Autodesk Fusion 360 part; units mm, degrees
(part 4 of 8)
  spline S1001 degree 3 poles (12.7984, -90.8958) (12.7866, -90.9224) (12.7444, -90.9476) (12.7042, -90.9476) knots 0 0 0 0 1 1 1 1
  spline S1002 degree 3 poles (12.7042, -90.9476) (12.6392, -90.9505) (12.642, -90.9527) (12.7088, -90.9646) knots 0 0 0 0 1 1 1 1
  spline S1003 degree 3 poles (14.8306, -88.329) (14.8946, -88.3388) (14.9475, -88.3398) (14.9491, -88.3321) knots 0 0 0 0 1 1 1 1
  spline S1004 degree 3 poles (14.9491, -88.3321) (14.9427, -88.3002) (14.7543, -88.2605) (14.7348, -88.2855) knots 0 0 0 0 1 1 1 1
  spline S1005 degree 3 poles (14.7348, -88.2855) (14.7218, -88.3022) (14.7666, -88.3193) (14.8306, -88.329) knots 0 0 0 0 1 1 1 1
  spline S1006 degree 3 poles (4.5302, -101.5016) (4.5488, -101.4892) (4.5748, -101.4559) (4.5845, -101.4321) knots 0 0 0 0 1 1 1 1
  spline S1007 degree 3 poles (4.5845, -101.4321) (4.5892, -101.4089) (4.5727, -101.4184) (4.5423, -101.4573) knots 0 0 0 0 1 1 1 1
  spline S1008 degree 3 poles (4.5423, -101.4573) (4.5119, -101.4963) (4.5066, -101.5145) (4.5302, -101.5016) knots 0 0 0 0 1 1 1 1
  spline S1009 degree 3 poles (11.2167, -93.0176) (11.2886, -92.9887) (11.3694, -92.931) (11.3998, -92.8921) knots 0 0 0 0 1 1 1 1
  spline S1010 degree 3 poles (11.3998, -92.8921) (11.4346, -92.8476) (11.3962, -92.8624) (11.2819, -92.9343) knots 0 0 0 0 1 1 1 1
  spline S1011 degree 3 poles (11.2819, -92.9343) (11.0653, -93.0739) (11.0544, -93.0878) (11.2167, -93.0176) knots 0 0 0 0 1 1 1 1
  spline S1012 degree 3 poles (12.0049, -91.9859) (11.9836, -92.0991) (12.0323, -92.1686) (12.1069, -92.1418) knots 0 0 0 0 1 1 1 1
  spline S1013 degree 3 poles (12.1069, -92.1418) (12.1333, -92.131) (12.1265, -92.1168) (12.0817, -92.0997) knots 0 0 0 0 1 1 1 1
  spline S1014 degree 3 poles (12.0817, -92.0997) (12.0291, -92.081) (12.0199, -92.0469) (12.038, -91.9492) knots 0 0 0 0 1 1 1 1
  spline S1015 degree 3 poles (12.038, -91.9492) (12.0549, -91.8818) (12.0566, -91.8338) (12.0435, -91.8505) knots 0 0 0 0 1 1 1 1
  spline S1016 degree 3 poles (12.0435, -91.8505) (12.0327, -91.8644) (12.0152, -91.9269) (12.0049, -91.9859) knots 0 0 0 0 1 1 1 1
  spline S1017 degree 3 poles (14.5723, -88.7227) (14.5927, -88.7252) (14.6175, -88.7221) (14.624, -88.7138) knots 0 0 0 0 1 1 1 1
  spline S1018 degree 3 poles (14.624, -88.7138) (14.6284, -88.7082) (14.6188, -88.6918) (14.6049, -88.681) knots 0 0 0 0 1 1 1 1
  spline S1019 degree 3 poles (14.6049, -88.681) (14.5882, -88.6679) (14.5662, -88.6731) (14.5532, -88.6898) knots 0 0 0 0 1 1 1 1
  spline S1020 degree 3 poles (14.5532, -88.6898) (14.5424, -88.7037) (14.5491, -88.718) (14.5723, -88.7227) knots 0 0 0 0 1 1 1 1
  spline S1021 degree 3 poles (4.281, -101.9695) (4.306, -101.989) (4.5908, -102.0772) (4.9108, -102.1661) knots 0 0 0 0 1 1 1 1
  spline S1022 degree 3 poles (4.9108, -102.1661) (5.4408, -102.3071) (5.533, -102.3209) (5.9897, -102.3151) knots 0 0 0 0 1 1 1 1
  line L78 (5.9897, -102.3151) -> (6.486, -102.3044)
  line L79 (6.486, -102.3044) -> (6.739, -102.502)
  line L80 (6.739, -102.502) -> (6.9892, -102.6975)
  line L81 (6.9892, -102.6975) -> (6.99, -105.5902)
  spline S1023 degree 3 poles (6.99, -105.5902) (6.9896, -107.1836) (6.9897, -108.5759) (6.9888, -108.6917) knots 0 0 0 0 1 1 1 1
  spline S1024 degree 3 poles (6.9888, -108.6917) (6.9873, -108.8024) (6.9877, -109.5011) (6.9879, -110.2399) knots 0 0 0 0 1 1 1 1
  spline S1025 degree 3 poles (6.9879, -110.2399) (6.9881, -110.9788) (6.991, -112.0868) (6.9887, -112.7028) knots 0 0 0 0 1 1 1 1
  spline S1026 degree 3 poles (6.9887, -112.7028) (6.9874, -115.455) (6.9879, -117.179) (6.9875, -118.3427) knots 0 0 0 0 1 1 1 1
  spline S1027 degree 3 poles (6.9875, -118.3427) (6.9869, -119.7703) (6.9887, -121.7907) (6.9896, -123.7836) knots 0 0 0 0 1 1 1 1
  spline S1028 degree 3 poles (6.9896, -123.7836) (6.9889, -124.5352) (6.9928, -125.1605) (7.0002, -125.1797) knots 0 0 0 0 1 1 1 1
  spline S1029 degree 3 poles (7.0002, -125.1797) (7.0128, -125.2209) (8.7969, -126.467) (8.9109, -126.5159) knots 0 0 0 0 1 1 1 1
  spline S1030 degree 3 poles (8.9109, -126.5159) (9.0544, -126.5787) (9.3568, -126.3807) (9.4107, -126.1856) knots 0 0 0 0 1 1 1 1
  spline S1031 degree 3 poles (9.4107, -126.1856) (9.4357, -126.1021) (9.4813, -126.0437) (9.6313, -125.9147) knots 0 0 0 0 1 1 1 1
  spline S1032 degree 3 poles (9.6313, -125.9147) (9.7355, -125.8215) (9.9286, -125.6545) (10.0551, -125.5385) knots 0 0 0 0 1 1 1 1
  spline S1033 degree 3 poles (10.0551, -125.5385) (10.2253, -125.3894) (10.2996, -125.3401) (10.3188, -125.3729) knots 0 0 0 0 1 1 1 1
  spline S1034 degree 3 poles (10.3188, -125.3729) (10.3502, -125.4243) (10.3645, -125.4175) (10.761, -125.0648) knots 0 0 0 0 1 1 1 1
  spline S1035 degree 3 poles (10.761, -125.0648) (11.0756, -124.7823) (11.1153, -124.7373) (11.2557, -124.4888) knots 0 0 0 0 1 1 1 1
  spline S1036 degree 3 poles (11.2557, -124.4888) (11.3514, -124.3263) (11.4189, -124.1596) (11.4315, -124.0576) knots 0 0 0 0 1 1 1 1
  spline S1037 degree 3 poles (11.4315, -124.0576) (11.4484, -123.9499) (11.5203, -123.7777) (11.6461, -123.5537) knots 0 0 0 0 1 1 1 1
  spline S1038 degree 3 poles (11.6461, -123.5537) (11.8113, -123.262) (11.8911, -123.1542) (12.2332, -122.7678) knots 0 0 0 0 1 1 1 1
  spline S1039 degree 3 poles (12.2332, -122.7678) (12.651, -122.3019) (12.7087, -122.1993) (12.6499, -122.0683) knots 0 0 0 0 1 1 1 1
  spline S1040 degree 3 poles (12.6499, -122.0683) (12.6364, -122.0398) (12.4699, -121.7485) (12.2816, -121.4223) knots 0 0 0 0 1 1 1 1
  spline S1041 degree 3 poles (12.2816, -121.4223) (12.0933, -121.0961) (11.9333, -120.7966) (11.9306, -120.7542) knots 0 0 0 0 1 1 1 1
  spline S1042 degree 3 poles (11.9306, -120.7542) (11.9279, -120.7118) (11.9034, -120.6344) (11.8763, -120.5774) knots 0 0 0 0 1 1 1 1
  spline S1043 degree 3 poles (11.8763, -120.5774) (11.8073, -120.425) (11.7691, -119.9296) (11.8234, -119.8601) knots 0 0 0 0 1 1 1 1
  spline S1044 degree 3 poles (11.8234, -119.8601) (11.8473, -119.8295) (12.0503, -119.6613) (12.2682, -119.4913) knots 0 0 0 0 1 1 1 1
  spline S1045 degree 3 poles (12.2682, -119.4913) (12.4861, -119.3213) (12.6847, -119.1587) (12.7086, -119.1281) knots 0 0 0 0 1 1 1 1
  spline S1046 degree 3 poles (12.7086, -119.1281) (12.7499, -119.0753) (12.7349, -118.871) (12.6848, -118.8319) knots 0 0 0 0 1 1 1 1
  spline S1047 degree 3 poles (12.6848, -118.8319) (12.6292, -118.7885) (12.0506, -117.8216) (12.0208, -117.7222) knots 0 0 0 0 1 1 1 1
  spline S1048 degree 3 poles (12.0208, -117.7222) (11.9944, -117.6299) (12.0202, -117.574) (12.3693, -116.9782) knots 0 0 0 0 1 1 1 1
  spline S1049 degree 3 poles (12.3693, -116.9782) (12.5773, -116.6259) (12.7532, -116.2977) (12.7604, -116.2541) knots 0 0 0 0 1 1 1 1
  spline S1050 degree 3 poles (12.7604, -116.2541) (12.7698, -116.2077) (12.7483, -116.1148) (12.7138, -116.0387) knots 0 0 0 0 1 1 1 1
  spline S1051 degree 3 poles (12.7138, -116.0387) (12.6217, -115.8414) (11.9083, -114.5542) (11.8777, -114.5303) knots 0 0 0 0 1 1 1 1
  spline S1052 degree 3 poles (11.8777, -114.5303) (11.8332, -114.4956) (11.8403, -114.3489) (11.8999, -113.9747) knots 0 0 0 0 1 1 1 1
  spline S1053 degree 3 poles (11.8999, -113.9747) (11.936, -113.7566) (11.9912, -113.5714) (12.0303, -113.5214) knots 0 0 0 0 1 1 1 1
  spline S1054 degree 3 poles (12.0303, -113.5214) (12.0672, -113.4741) (12.3083, -113.3088) (12.5611, -113.1571) knots 0 0 0 0 1 1 1 1
  spline S1055 degree 3 poles (12.5611, -113.1571) (12.8161, -113.0027) (13.0419, -112.8568) (13.0637, -112.829) knots 0 0 0 0 1 1 1 1
  spline S1056 degree 3 poles (13.0637, -112.829) (13.1223, -112.754) (13.1248, -112.5903) (13.0742, -112.1165) knots 0 0 0 0 1 1 1 1
  line L82 (13.0742, -112.1165) -> (13.0312, -111.6844)
  line L83 (13.0312, -111.6844) -> (12.759, -111.2077)
  spline S1057 degree 3 poles (12.759, -111.2077) (12.4924, -110.7352) (12.489, -110.7281) (12.4214, -110.2589) knots 0 0 0 0 1 1 1 1
  spline S1058 degree 3 poles (12.4214, -110.2589) (12.3842, -109.9971) (12.3686, -109.7477) (12.3885, -109.705) knots 0 0 0 0 1 1 1 1
  spline S1059 degree 3 poles (12.3885, -109.705) (12.41, -109.6546) (12.5476, -109.5472) (12.7505, -109.4193) knots 0 0 0 0 1 1 1 1
  spline S1060 degree 3 poles (12.7505, -109.4193) (13.1329, -109.1763) (13.1565, -109.1231) (13.0008, -108.8985) knots 0 0 0 0 1 1 1 1
  spline S1061 degree 3 poles (13.0008, -108.8985) (12.9486, -108.8219) (12.7984, -108.6016) (12.6667, -108.4092) knots 0 0 0 0 1 1 1 1
  spline S1062 degree 3 poles (12.6667, -108.4092) (12.5329, -108.2195) (12.4166, -108.0302) (12.4068, -107.9912) knots 0 0 0 0 1 1 1 1
  spline S1063 degree 3 poles (12.4068, -107.9912) (12.3832, -107.9011) (12.3853, -106.6493) (12.4092, -106.6187) knots 0 0 0 0 1 1 1 1
  spline S1064 degree 3 poles (12.4092, -106.6187) (12.4179, -106.6076) (12.442, -106.5996) (12.4603, -106.6049) knots 0 0 0 0 1 1 1 1
  spline S1065 degree 3 poles (12.4603, -106.6049) (12.5206, -106.6251) (13.1255, -106.6187) (13.1428, -106.5965) knots 0 0 0 0 1 1 1 1
  spline S1066 degree 3 poles (13.1428, -106.5965) (13.1581, -106.577) (13.1685, -105.4749) (13.1578, -104.4458) knots 0 0 0 0 1 1 1 1
  spline S1067 degree 3 poles (13.1578, -104.4458) (13.159, -104.1692) (13.1651, -103.9322) (13.1781, -103.9155) knots 0 0 0 0 1 1 1 1
  spline S1068 degree 3 poles (13.1781, -103.9155) (13.1911, -103.8989) (13.2019, -103.6387) (13.2023, -103.3345) knots 0 0 0 0 1 1 1 1
  spline S1069 degree 3 poles (13.2023, -103.3345) (13.1977, -103.031) (13.2023, -102.7615) (13.1992, -102.7367) knots 0 0 0 0 1 1 1 1
  spline S1070 degree 3 poles (13.1992, -102.7367) (13.2015, -102.6937) (13.5834, -102.3654) (13.6673, -102.3324) knots 0 0 0 0 1 1 1 1
  spline S1071 degree 3 poles (13.6673, -102.3324) (13.6915, -102.3245) (13.9245, -102.3185) (14.1862, -102.3215) knots 0 0 0 0 1 1 1 1
  spline S1072 degree 3 poles (14.1862, -102.3215) (14.6067, -102.3277) (14.7228, -102.3109) (15.2748, -102.1602) knots 0 0 0 0 1 1 1 1
  spline S1073 degree 3 poles (15.2748, -102.1602) (15.6125, -102.066) (15.9073, -101.9694) (15.9241, -101.9423) knots 0 0 0 0 1 1 1 1
  spline S1074 degree 3 poles (15.9241, -101.9423) (15.9545, -101.9033) (15.9489, -101.899) (15.9117, -101.9237) knots 0 0 0 0 1 1 1 1
  spline S1075 degree 3 poles (15.9117, -101.9237) (15.8832, -101.9372) (15.6092, -102.0186) (15.2956, -102.1049) knots 0 0 0 0 1 1 1 1
  spline S1076 degree 3 poles (15.2956, -102.1049) (14.804, -102.2356) (14.6632, -102.2554) (14.2136, -102.2578) knots 0 0 0 0 1 1 1 1
  spline S1077 degree 3 poles (14.2136, -102.2578) (13.7436, -102.2577) (13.5797, -102.2326) (13.7682, -102.1919) knots 0 0 0 0 1 1 1 1
  spline S1078 degree 3 poles (13.7682, -102.1919) (13.8391, -102.1756) (13.8363, -102.1735) (13.7546, -102.1634) knots 0 0 0 0 1 1 1 1
  spline S1079 degree 3 poles (13.7546, -102.1634) (13.6863, -102.1592) (13.6649, -102.1694) (13.6654, -102.2146) knots 0 0 0 0 1 1 1 1
  spline S1080 degree 3 poles (13.6654, -102.2146) (13.6668, -102.2873) (13.2945, -102.5918) (13.1769, -102.6163) knots 0 0 0 0 1 1 1 1
  spline S1081 degree 3 poles (13.1769, -102.6163) (13.1104, -102.627) (13.1001, -102.6459) (13.107, -102.7632) knots 0 0 0 0 1 1 1 1
  spline S1082 degree 3 poles (13.107, -102.7632) (13.1289, -103.0847) (13.111, -103.8811) (13.0881, -103.8989) knots 0 0 0 0 1 1 1 1
  spline S1083 degree 3 poles (13.0881, -103.8989) (13.0695, -103.9113) (13.0342, -103.9106) (13.0055, -103.9016) knots 0 0 0 0 1 1 1 1
  spline S1084 degree 3 poles (13.0055, -103.9016) (12.9634, -103.8866) (12.9699, -103.8783) (13.0408, -103.862) knots 0 0 0 0 1 1 1 1
  spline S1085 degree 3 poles (13.0408, -103.862) (13.1188, -103.8424) (13.1188, -103.8424) (13.0461, -103.8438) knots 0 0 0 0 1 1 1 1
  spline S1086 degree 3 poles (13.0461, -103.8438) (13.0031, -103.8415) (12.9675, -103.8585) (12.9622, -103.8767) knots 0 0 0 0 1 1 1 1
  spline S1087 degree 3 poles (12.9622, -103.8767) (12.9619, -103.8943) (12.5995, -103.9112) (12.1592, -103.9074) knots 0 0 0 0 1 1 1 1
  spline S1088 degree 3 poles (12.1592, -103.9074) (11.7168, -103.9065) (11.3566, -103.9205) (11.3569, -103.9431) knots 0 0 0 0 1 1 1 1
  spline S1089 degree 3 poles (11.3569, -103.9431) (11.3593, -103.9629) (11.351, -103.9564) (11.3402, -103.9301) knots 0 0 0 0 1 1 1 1
  spline S1090 degree 3 poles (11.3402, -103.9301) (11.3226, -103.8895) (11.3384, -103.875) (11.4149, -103.8631) knots 0 0 0 0 1 1 1 1
  spline S1091 degree 3 poles (11.4149, -103.8631) (11.5084, -103.8466) (11.5078, -103.8417) (11.4311, -103.831) knots 0 0 0 0 1 1 1 1
  spline S1092 degree 3 poles (11.4311, -103.831) (11.3896, -103.821) (11.3048, -103.8264) (11.2482, -103.8358) knots 0 0 0 0 1 1 1 1
  spline S1093 degree 3 poles (11.2482, -103.8358) (11.1575, -103.8545) (11.1553, -103.8573) (11.2231, -103.8565) knots 0 0 0 0 1 1 1 1
  spline S1094 degree 3 poles (11.2231, -103.8565) (11.2936, -103.8579) (11.3047, -103.8666) (11.2981, -103.9152) knots 0 0 0 0 1 1 1 1
  spline S1095 degree 3 poles (11.2981, -103.9152) (11.2947, -103.9483) (11.2807, -103.9776) (11.2686, -103.9816) knots 0 0 0 0 1 1 1 1
  spline S1096 degree 3 poles (11.2686, -103.9816) (11.2543, -103.9884) (11.259, -104.0054) (11.2812, -104.0228) knots 0 0 0 0 1 1 1 1
  spline S1097 degree 3 poles (11.2812, -104.0228) (11.3034, -104.0402) (11.3232, -104.0377) (11.3258, -104.0173) knots 0 0 0 0 1 1 1 1
  spline S1098 degree 3 poles (11.3258, -104.0173) (11.3261, -103.9997) (11.3404, -103.9929) (11.3543, -104.0038) knots 0 0 0 0 1 1 1 1
  spline S1099 degree 3 poles (11.3543, -104.0038) (11.3682, -104.0146) (11.3806, -104.1363) (11.3794, -104.2696) knots 0 0 0 0 1 1 1 1
  spline S1100 degree 3 poles (11.3794, -104.2696) (11.3767, -104.4735) (11.3646, -104.5177) (11.3107, -104.5294) knots 0 0 0 0 1 1 1 1
  spline S1101 degree 3 poles (11.3107, -104.5294) (11.264, -104.5376) (11.2531, -104.5515) (11.2754, -104.5689) knots 0 0 0 0 1 1 1 1
  spline S1102 degree 3 poles (11.2754, -104.5689) (11.292, -104.5819) (11.3168, -104.5789) (11.3298, -104.5622) knots 0 0 0 0 1 1 1 1
  spline S1103 degree 3 poles (11.3298, -104.5622) (11.3841, -104.4927) (11.3825, -104.2541) (11.3803, -109.6604) knots 0 0 0 0 1 1 1 1
  spline S1104 degree 3 poles (11.3803, -109.6604) (11.378, -111.136) (11.3595, -112.1109) (11.3328, -112.1393) knots 0 0 0 0 1 1 1 1
  spline S1105 degree 3 poles (11.3328, -112.1393) (11.3033, -112.1655) (11.3036, -112.1881) (11.3324, -112.1971) knots 0 0 0 0 1 1 1 1
  spline S1106 degree 3 poles (11.3324, -112.1971) (11.3611, -112.2062) (11.3792, -112.7217) (11.3792, -113.541) knots 0 0 0 0 1 1 1 1
  line L84 (11.3792, -113.541) -> (11.3813, -114.8677)
  line L85 (11.3813, -114.8677) -> (11.2739, -114.8734)
  line L86 (11.2739, -114.8734) -> (11.1715, -114.8784)
  line L87 (11.1715, -114.8784) -> (11.2736, -114.891)
  spline S1107 degree 3 poles (11.2736, -114.891) (11.3729, -114.9014) (11.379, -114.9107) (11.3784, -115.049) knots 0 0 0 0 1 1 1 1
  spline S1108 degree 3 poles (11.3784, -115.049) (11.3782, -115.1295) (11.3789, -115.6672) (11.3795, -116.2452) knots 0 0 0 0 1 1 1 1
  spline S1109 degree 3 poles (11.3795, -116.2452) (11.3773, -116.821) (11.3759, -117.3213) (11.3796, -117.351) knots 0 0 0 0 1 1 1 1
  spline S1110 degree 3 poles (11.3796, -117.351) (11.3767, -117.3891) (11.3522, -117.4147) (11.3033, -117.4257) knots 0 0 0 0 1 1 1 1
  spline S1111 degree 3 poles (11.3033, -117.4257) (11.2324, -117.442) (11.233, -117.4469) (11.3008, -117.4462) knots 0 0 0 0 1 1 1 1
  spline S1112 degree 3 poles (11.3008, -117.4462) (11.3834, -117.4436) (11.3849, -117.4761) (11.3791, -118.9847) knots 0 0 0 0 1 1 1 1
  spline S1113 degree 3 poles (11.3791, -118.9847) (11.377, -119.6635) (11.3693, -119.8052) (11.33, -119.6492) knots 0 0 0 0 1 1 1 1
  spline S1114 degree 3 poles (11.33, -119.6492) (11.3184, -119.5953) (11.3122, -119.5861) (11.3072, -119.6269) knots 0 0 0 0 1 1 1 1
  spline S1115 degree 3 poles (11.3072, -119.6269) (11.3031, -119.655) (11.2693, -119.6868) (11.2275, -119.6945) knots 0 0 0 0 1 1 1 1
  spline S1116 degree 3 poles (11.2275, -119.6945) (11.1665, -119.7095) (11.1693, -119.7117) (11.2658, -119.7199) knots 0 0 0 0 1 1 1 1
  spline S1117 degree 3 poles (11.2658, -119.7199) (11.3982, -119.7338) (11.3837, -119.5748) (11.3812, -121.171) knots 0 0 0 0 1 1 1 1
  spline S1118 degree 3 poles (11.3812, -121.171) (11.379, -121.7468) (11.3803, -122.2493) (11.3796, -122.2845) knots 0 0 0 0 1 1 1 1
  spline S1119 degree 3 poles (11.3796, -122.2845) (11.3786, -122.3374) (11.3737, -122.3381) (11.3456, -122.2937) knots 0 0 0 0 1 1 1 1
  spline S1120 degree 3 poles (11.3456, -122.2937) (11.3209, -122.2566) (11.3082, -122.2556) (11.2955, -122.2949) knots 0 0 0 0 1 1 1 1
  spline S1121 degree 3 poles (11.2955, -122.2949) (11.2864, -122.3236) (11.3006, -122.3571) (11.3278, -122.3738) knots 0 0 0 0 1 1 1 1
  spline S1122 degree 3 poles (11.3278, -122.3738) (11.376, -122.3981) (11.3855, -122.701) (11.3735, -123.7078) knots 0 0 0 0 1 1 1 1
  spline S1123 degree 3 poles (11.3735, -123.7078) (11.3706, -124.0324) (11.3542, -124.145) (11.2887, -124.246) knots 0 0 0 0 1 1 1 1
  spline S1124 degree 3 poles (11.2887, -124.246) (11.2471, -124.3164) (11.172, -124.4413) (11.1223, -124.5278) knots 0 0 0 0 1 1 1 1
  spline S1125 degree 3 poles (11.1223, -124.5278) (11.0338, -124.687) (10.5314, -125.1809) (10.4119, -125.2308) knots 0 0 0 0 1 1 1 1
  spline S1126 degree 3 poles (10.4119, -125.2308) (10.3664, -125.2489) (10.3553, -125.0568) (10.359, -124.3702) knots 0 0 0 0 1 1 1 1
  spline S1127 degree 3 poles (10.359, -124.3702) (10.3595, -123.8826) (10.3618, -123.2263) (10.3609, -122.9123) knots 0 0 0 0 1 1 1 1
  spline S1128 degree 3 poles (10.3609, -122.9123) (10.3629, -122.4571) (10.3786, -122.3396) (10.4244, -122.344) knots 0 0 0 0 1 1 1 1
  spline S1129 degree 3 poles (10.4244, -122.344) (10.4723, -122.3457) (10.4717, -122.3407) (10.4257, -122.3137) knots 0 0 0 0 1 1 1 1
  spline S1130 degree 3 poles (10.4257, -122.3137) (10.3796, -122.2867) (10.3639, -121.688) (10.364, -119.6824) knots 0 0 0 0 1 1 1 1
  spline S1131 degree 3 poles (10.364, -119.6824) (10.3625, -115.1059) (10.3617, -114.8949) (10.4038, -114.9099) knots 0 0 0 0 1 1 1 1
  spline S1132 degree 3 poles (10.4038, -114.9099) (10.4591, -114.9307) (10.484, -114.8874) (10.4497, -114.8338) knots 0 0 0 0 1 1 1 1
  spline S1133 degree 3 poles (10.4497, -114.8338) (10.4278, -114.7988) (10.4158, -114.8028) (10.4008, -114.8449) knots 0 0 0 0 1 1 1 1
  spline S1134 degree 3 poles (10.4008, -114.8449) (10.3821, -114.8974) (10.3794, -114.8953) (10.3715, -114.8309) knots 0 0 0 0 1 1 1 1
  spline S1135 degree 3 poles (10.3715, -114.8309) (10.3401, -114.596) (10.3688, -112.2099) (10.4017, -112.1908) knots 0 0 0 0 1 1 1 1
  spline S1136 degree 3 poles (10.4017, -112.1908) (10.4224, -112.1757) (10.425, -112.1552) (10.4033, -112.1428) knots 0 0 0 0 1 1 1 1
  spline S1137 degree 3 poles (10.4033, -112.1428) (10.3811, -112.1254) (10.364, -111.454) (10.363, -110.6474) knots 0 0 0 0 1 1 1 1
  line L88 (10.363, -110.6474) -> (10.3609, -109.1774)
  line L89 (10.3609, -109.1774) -> (10.4683, -109.1717)
  line L90 (10.4683, -109.1717) -> (10.5757, -109.1661)
  line L91 (10.5757, -109.1661) -> (10.4686, -109.1541)
  line L92 (10.4686, -109.1541) -> (10.3638, -109.1393)
  line L93 (10.3638, -109.1393) -> (10.3631, -107.8853)
  spline S1138 degree 3 poles (10.3631, -107.8853) (10.3634, -107.1916) (10.3826, -106.6112) (10.3978, -106.5917) knots 0 0 0 0 1 1 1 1
  spline S1139 degree 3 poles (10.3978, -106.5917) (10.418, -106.5717) (10.4177, -106.5491) (10.3988, -106.5388) knots 0 0 0 0 1 1 1 1
  spline S1140 degree 3 poles (10.3988, -106.5388) (10.3828, -106.5307) (10.3661, -106.0879) (10.3639, -105.5579) knots 0 0 0 0 1 1 1 1
  spline S1141 degree 3 poles (10.3639, -105.5579) (10.3642, -104.9673) (10.3449, -104.5851) (10.3156, -104.5711) knots 0 0 0 0 1 1 1 1
  spline S1142 degree 3 poles (10.3156, -104.5711) (10.289, -104.5593) (10.2782, -104.533) (10.2912, -104.5163) knots 0 0 0 0 1 1 1 1
  spline S1143 degree 3 poles (10.2912, -104.5163) (10.3043, -104.4996) (10.3197, -104.5028) (10.3299, -104.5241) knots 0 0 0 0 1 1 1 1
  spline S1144 degree 3 poles (10.3299, -104.5241) (10.3373, -104.5433) (10.3555, -104.5486) (10.3664, -104.5347) knots 0 0 0 0 1 1 1 1
  spline S1145 degree 3 poles (10.3664, -104.5347) (10.3794, -104.518) (10.4042, -104.515) (10.4209, -104.528) knots 0 0 0 0 1 1 1 1
  spline S1146 degree 3 poles (10.4209, -104.528) (10.4348, -104.5389) (10.4344, -104.5565) (10.4152, -104.5639) knots 0 0 0 0 1 1 1 1
  spline S1147 degree 3 poles (10.4152, -104.5639) (10.3356, -104.5913) (10.4401, -104.6639) (10.5335, -104.6474) knots 0 0 0 0 1 1 1 1
  spline S1148 degree 3 poles (10.5335, -104.6474) (10.6314, -104.6253) (10.6314, -104.6253) (10.5339, -104.6298) knots 0 0 0 0 1 1 1 1
  spline S1149 degree 3 poles (10.5339, -104.6298) (10.4463, -104.633) (10.438, -104.6265) (10.4545, -104.5767) knots 0 0 0 0 1 1 1 1
  spline S1150 degree 3 poles (10.4545, -104.5767) (10.4794, -104.4932) (10.4269, -104.4745) (10.226, -104.4967) knots 0 0 0 0 1 1 1 1
  spline S1151 degree 3 poles (10.226, -104.4967) (10.127, -104.5088) (10.0901, -104.5159) (10.148, -104.5163) knots 0 0 0 0 1 1 1 1
  spline S1152 degree 3 poles (10.148, -104.5163) (10.2031, -104.5146) (10.2522, -104.5261) (10.2541, -104.541) knots 0 0 0 0 1 1 1 1
  spline S1153 degree 3 poles (10.2541, -104.541) (10.2559, -104.5558) (10.0841, -104.5694) (9.8753, -104.5674) knots 0 0 0 0 1 1 1 1
  spline S1154 degree 3 poles (9.8753, -104.5674) (9.5965, -104.5689) (9.4876, -104.5823) (9.4705, -104.6271) knots 0 0 0 0 1 1 1 1
  spline S1155 degree 3 poles (9.4705, -104.6271) (9.454, -104.6769) (9.449, -104.6775) (9.4522, -104.6218) knots 0 0 0 0 1 1 1 1
  spline S1156 degree 3 poles (9.4522, -104.6218) (9.456, -104.5711) (9.4421, -104.5602) (9.3926, -104.5663) knots 0 0 0 0 1 1 1 1
  spline S1157 degree 3 poles (9.3926, -104.5663) (9.3629, -104.57) (9.3221, -104.5649) (9.3082, -104.5541) knots 0 0 0 0 1 1 1 1
  spline S1158 degree 3 poles (9.3082, -104.5541) (9.2943, -104.5432) (9.3652, -104.527) (9.467, -104.517) knots 0 0 0 0 1 1 1 1
  spline S1159 degree 3 poles (9.467, -104.517) (9.5716, -104.5092) (9.6029, -104.4978) (9.5422, -104.4952) knots 0 0 0 0 1 1 1 1
  spline S1160 degree 3 poles (9.5422, -104.4952) (9.4766, -104.4932) (9.3878, -104.4865) (9.3399, -104.4848) knots 0 0 0 0 1 1 1 1
  spline S1161 degree 3 poles (9.3399, -104.4848) (9.2638, -104.4791) (9.2551, -104.4902) (9.2602, -104.5524) knots 0 0 0 0 1 1 1 1
  spline S1162 degree 3 poles (9.2602, -104.5524) (9.2675, -104.6118) (9.2567, -104.6257) (9.2006, -104.6402) knots 0 0 0 0 1 1 1 1
  spline S1163 degree 3 poles (9.2006, -104.6402) (9.1369, -104.653) (9.1396, -104.6552) (9.2235, -104.6625) knots 0 0 0 0 1 1 1 1
  spline S1164 degree 3 poles (9.2235, -104.6625) (9.2875, -104.6722) (9.311, -104.6593) (9.2969, -104.6258) knots 0 0 0 0 1 1 1 1
  spline S1165 degree 3 poles (9.2969, -104.6258) (9.2849, -104.5896) (9.2892, -104.584) (9.3143, -104.6036) knots 0 0 0 0 1 1 1 1
  spline S1166 degree 3 poles (9.3143, -104.6036) (9.3337, -104.6188) (9.3498, -105.0566) (9.3486, -105.5795) knots 0 0 0 0 1 1 1 1
  line L94 (9.3486, -105.5795) -> (9.3518, -106.5266)
  line L95 (9.3518, -106.5266) -> (9.2088, -106.5492)
  line L96 (9.2088, -106.5492) -> (9.0658, -106.5718)
  line L97 (9.0658, -106.5718) -> (9.2075, -106.5795)
  spline S1167 degree 3 poles (9.2075, -106.5795) (9.2929, -106.5791) (9.3483, -106.6) (9.3519, -106.6297) knots 0 0 0 0 1 1 1 1
  spline S1168 degree 3 poles (9.3519, -106.6297) (9.3522, -106.6523) (9.3516, -107.2203) (9.3532, -107.8887) knots 0 0 0 0 1 1 1 1
  spline S1169 degree 3 poles (9.3532, -107.8887) (9.35, -108.9069) (9.3375, -109.112) (9.2827, -109.1363) knots 0 0 0 0 1 1 1 1
  spline S1170 degree 3 poles (9.2827, -109.1363) (9.2328, -109.1601) (9.2248, -109.1761) (9.2526, -109.1978) knots 0 0 0 0 1 1 1 1
  spline S1171 degree 3 poles (9.2526, -109.1978) (9.2748, -109.2152) (9.2946, -109.2128) (9.2971, -109.1924) knots 0 0 0 0 1 1 1 1
  spline S1172 degree 3 poles (9.2971, -109.1924) (9.2975, -109.1747) (9.3117, -109.168) (9.3256, -109.1788) knots 0 0 0 0 1 1 1 1
  spline S1173 degree 3 poles (9.3256, -109.1788) (9.3451, -109.194) (9.3588, -110.8611) (9.3473, -111.8729) knots 0 0 0 0 1 1 1 1
  spline S1174 degree 3 poles (9.3473, -111.8729) (9.3448, -112.1396) (9.3417, -112.155) (9.2613, -112.1549) knots 0 0 0 0 1 1 1 1
  spline S1175 degree 3 poles (9.2613, -112.1549) (9.1836, -112.1569) (9.1836, -112.1569) (9.2637, -112.1747) knots 0 0 0 0 1 1 1 1
  spline S1176 degree 3 poles (9.2637, -112.1747) (9.3438, -112.1925) (9.3487, -112.2321) (9.3495, -112.6894) knots 0 0 0 0 1 1 1 1
  spline S1177 degree 3 poles (9.3495, -112.6894) (9.3526, -112.9605) (9.3701, -113.1845) (9.3955, -113.1864) knots 0 0 0 0 1 1 1 1
  spline S1178 degree 3 poles (9.3955, -113.1864) (9.4187, -113.1911) (9.4171, -113.1988) (9.3929, -113.2068) knots 0 0 0 0 1 1 1 1
  spline S1179 degree 3 poles (9.3929, -113.2068) (9.3688, -113.2148) (9.3504, -113.5765) (9.3506, -114.0288) knots 0 0 0 0 1 1 1 1
  spline S1180 degree 3 poles (9.3506, -114.0288) (9.3496, -114.798) (9.3393, -114.9601) (9.3016, -114.7964) knots 0 0 0 0 1 1 1 1
  spline S1181 degree 3 poles (9.3016, -114.7964) (9.2888, -114.7326) (9.2844, -114.7382) (9.2762, -114.8347) knots 0 0 0 0 1 1 1 1
  spline S1182 degree 3 poles (9.2762, -114.8347) (9.2644, -114.9643) (9.2786, -114.9977) (9.3035, -114.9143) knots 0 0 0 0 1 1 1 1
  spline S1183 degree 3 poles (9.3035, -114.9143) (9.3098, -114.8833) (9.325, -114.8639) (9.3333, -114.8704) knots 0 0 0 0 1 1 1 1
  spline S1184 degree 3 poles (9.3333, -114.8704) (9.3417, -114.8769) (9.3491, -115.5722) (9.3522, -116.4162) knots 0 0 0 0 1 1 1 1
  spline S1185 degree 3 poles (9.3522, -116.4162) (9.3504, -117.2609) (9.3514, -118.9271) (9.3519, -120.1183) knots 0 0 0 0 1 1 1 1
  spline S1186 degree 3 poles (9.3519, -120.1183) (9.3524, -121.3095) (9.3351, -122.2943) (9.3115, -122.3073) knots 0 0 0 0 1 1 1 1
  spline S1187 degree 3 poles (9.3115, -122.3073) (9.2908, -122.3224) (9.2882, -122.3428) (9.3099, -122.3552) knots 0 0 0 0 1 1 1 1
  spline S1188 degree 3 poles (9.3099, -122.3552) (9.3426, -122.3763) (9.3633, -124.7965) (9.3459, -125.9648) knots 0 0 0 0 1 1 1 1
  spline S1189 degree 3 poles (9.3459, -125.9648) (9.3418, -126.1765) (9.3252, -126.2665) (9.299, -126.1968) knots 0 0 0 0 1 1 1 1
  spline S1190 degree 3 poles (9.299, -126.1968) (9.2922, -126.1825) (9.2563, -126.2171) (9.2162, -126.2798) knots 0 0 0 0 1 1 1 1
  spline S1191 degree 3 poles (9.2162, -126.2798) (9.115, -126.438) (8.9819, -126.4594) (8.8126, -126.3495) knots 0 0 0 0 1 1 1 1
  spline S1192 degree 3 poles (8.8126, -126.3495) (8.7366, -126.3035) (8.4178, -126.0813) (8.0989, -125.8591) knots 0 0 0 0 1 1 1 1
  spline S1193 degree 3 poles (8.0989, -125.8591) (7.7801, -125.6368) (7.4202, -125.387) (7.2991, -125.3013) knots 0 0 0 0 1 1 1 1
  spline S1194 degree 3 poles (7.2991, -125.3013) (7.0964, -125.1654) (7.0785, -125.1424) (7.0719, -125.0477) knots 0 0 0 0 1 1 1 1
  spline S1195 degree 3 poles (7.0719, -125.0477) (7.0696, -124.9877) (7.0699, -124.4373) (7.0727, -123.8262) knots 0 0 0 0 1 1 1 1
  spline S1196 degree 3 poles (7.0727, -123.8262) (7.075, -123.2102) (7.0744, -122.6322) (7.0755, -122.5391) knots 0 0 0 0 1 1 1 1
  line L98 (7.0755, -122.5391) -> (7.0747, -122.3683)
  line L99 (7.0747, -122.3683) -> (7.2, -122.3453)
  line L100 (7.2, -122.3453) -> (7.3254, -122.3224)
  line L101 (7.3254, -122.3224) -> (7.2032, -122.3299)
  line L102 (7.2032, -122.3299) -> (7.0809, -122.3374)
  line L103 (7.0809, -122.3374) -> (7.0775, -121.9407)
  spline S1197 degree 3 poles (7.0775, -121.9407) (7.0761, -121.7247) (7.0773, -121.1616) (7.0752, -120.6944) knots 0 0 0 0 1 1 1 1
  spline S1198 degree 3 poles (7.0752, -120.6944) (7.0781, -120.2266) (7.0784, -119.8194) (7.0747, -119.7897) knots 0 0 0 0 1 1 1 1
  spline S1199 degree 3 poles (7.0747, -119.7897) (7.0776, -119.7516) (7.1021, -119.726) (7.151, -119.715) knots 0 0 0 0 1 1 1 1
  spline S1200 degree 3 poles (7.151, -119.715) (7.2191, -119.6966) (7.2213, -119.6938) (7.1585, -119.6939) knots 0 0 0 0 1 1 1 1
  spline S1201 degree 3 poles (7.1585, -119.6939) (7.0681, -119.695) (7.0716, -119.8051) (7.0753, -117.8293) knots 0 0 0 0 1 1 1 1
  spline S1202 degree 3 poles (7.0753, -117.8293) (7.0764, -116.9168) (7.0767, -115.8964) (7.075, -115.5548) knots 0 0 0 0 1 1 1 1
  spline S1203 degree 3 poles (7.075, -115.5548) (7.0739, -115.2182) (7.0788, -114.9311) (7.0875, -114.9199) knots 0 0 0 0 1 1 1 1
  spline S1204 degree 3 poles (7.0875, -114.9199) (7.094, -114.9116) (7.0947, -114.8763) (7.0855, -114.8423) knots 0 0 0 0 1 1 1 1
  spline S1205 degree 3 poles (7.0855, -114.8423) (7.0791, -114.8104) (7.0728, -114.3085) (7.075, -113.7327) knots 0 0 0 0 1 1 1 1
  spline S1206 degree 3 poles (7.075, -113.7327) (7.0744, -113.1547) (7.0753, -112.569) (7.0766, -112.4357) knots 0 0 0 0 1 1 1 1
  spline S1207 degree 3 poles (7.0766, -112.4357) (7.0748, -112.2374) (7.0864, -112.1882) (7.1424, -112.1738) knots 0 0 0 0 1 1 1 1
  spline S1208 degree 3 poles (7.1424, -112.1738) (7.1984, -112.1593) (7.1984, -112.1593) (7.1406, -112.1589) knots 0 0 0 0 1 1 1 1
  spline S1209 degree 3 poles (7.1406, -112.1589) (7.0849, -112.1557) (7.0746, -111.9283) (7.0729, -110.7271) knots 0 0 0 0 1 1 1 1
  spline S1210 degree 3 poles (7.0729, -110.7271) (7.0715, -109.9381) (7.0742, -109.2643) (7.082, -109.2256) knots 0 0 0 0 1 1 1 1
  spline S1211 degree 3 poles (7.082, -109.2256) (7.0849, -109.1875) (7.0859, -109.1346) (7.0823, -109.1049) knots 0 0 0 0 1 1 1 1
  spline S1212 degree 3 poles (7.0823, -109.1049) (7.0746, -109.0631) (7.07, -107.6538) (7.0738, -106.7435) knots 0 0 0 0 1 1 1 1
  spline S1213 degree 3 poles (7.0738, -106.7435) (7.0753, -106.6327) (7.0741, -106.0498) (7.0738, -105.4542) knots 0 0 0 0 1 1 1 1
  spline S1214 degree 3 poles (7.0738, -105.4542) (7.0719, -103.8007) (7.0683, -103.8741) (7.1491, -103.8566) knots 0 0 0 0 1 1 1 1
  spline S1215 degree 3 poles (7.1491, -103.8566) (7.2073, -103.8394) (7.2073, -103.8394) (7.1445, -103.8396) knots 0 0 0 0 1 1 1 1
  spline S1216 degree 3 poles (7.1445, -103.8396) (7.0839, -103.837) (7.072, -103.7605) (7.0728, -103.2553) knots 0 0 0 0 1 1 1 1
  spline S1217 degree 3 poles (7.0728, -103.2553) (7.0713, -102.9362) (7.0886, -102.6677) (7.11, -102.6576) knots 0 0 0 0 1 1 1 1
  spline S1218 degree 3 poles (7.11, -102.6576) (7.1313, -102.6474) (7.1224, -102.6359) (7.0936, -102.6269) knots 0 0 0 0 1 1 1 1
  spline S1219 degree 3 poles (7.0936, -102.6269) (7.0621, -102.6157) (7.0274, -102.6199) (7.0166, -102.6338) knots 0 0 0 0 1 1 1 1
  spline S1220 degree 3 poles (7.0166, -102.6338) (7.0057, -102.6477) (6.8803, -102.5676) (6.7385, -102.4569) knots 0 0 0 0 1 1 1 1
  line L104 (6.7385, -102.4569) -> (6.4827, -102.2571)
  line L105 (6.4827, -102.2571) -> (5.9951, -102.2566)
  spline S1221 degree 3 poles (5.9951, -102.2566) (5.5251, -102.2565) (5.3463, -102.2332) (5.5503, -102.1956) knots 0 0 0 0 1 1 1 1
  spline S1222 degree 3 poles (5.5503, -102.1956) (5.6509, -102.1757) (5.6509, -102.1757) (5.5593, -102.1669) knots 0 0 0 0 1 1 1 1
  spline S1223 degree 3 poles (5.5593, -102.1669) (5.508, -102.1581) (5.4548, -102.1747) (5.4429, -102.2013) knots 0 0 0 0 1 1 1 1
  spline S1224 degree 3 poles (5.4429, -102.2013) (5.4181, -102.2445) (5.1602, -102.1907) (4.4885, -102.0018) knots 0 0 0 0 1 1 1 1
  spline S1225 degree 3 poles (4.4885, -102.0018) (4.3454, -101.9615) (4.2532, -101.9477) (4.281, -101.9695) knots 0 0 0 0 1 1 1 1
  spline S1226 degree 3 poles (9.5212, -104.631) (9.5308, -104.6072) (9.5621, -104.5958) (9.5909, -104.6048) knots 0 0 0 0 1 1 1 1
  spline S1227 degree 3 poles (9.5909, -104.6048) (9.6196, -104.6138) (9.6214, -104.6287) (9.5951, -104.6395) knots 0 0 0 0 1 1 1 1
  spline S1228 degree 3 poles (9.5951, -104.6395) (9.5276, -104.6628) (9.5669, -104.6756) (9.6499, -104.6554) knots 0 0 0 0 1 1 1 1
  spline S1229 degree 3 poles (9.6499, -104.6554) (9.7158, -104.6397) (9.718, -104.637) (9.6644, -104.631) knots 0 0 0 0 1 1 1 1
  spline S1230 degree 3 poles (9.6644, -104.631) (9.6109, -104.625) (9.6131, -104.6222) (9.679, -104.6066) knots 0 0 0 0 1 1 1 1
  spline S1231 degree 3 poles (9.679, -104.6066) (9.7571, -104.5869) (9.8312, -104.618) (9.7665, -104.6436) knots 0 0 0 0 1 1 1 1
  spline S1232 degree 3 poles (9.7665, -104.6436) (9.6969, -104.6697) (9.7454, -104.6763) (9.851, -104.6558) knots 0 0 0 0 1 1 1 1
  spline S1233 degree 3 poles (9.851, -104.6558) (9.9516, -104.6359) (9.9537, -104.6331) (9.8656, -104.6314) knots 0 0 0 0 1 1 1 1
  spline S1234 degree 3 poles (9.8656, -104.6314) (9.7774, -104.6297) (9.7796, -104.6269) (9.8802, -104.607) knots 0 0 0 0 1 1 1 1
  spline S1235 degree 3 poles (9.8802, -104.607) (9.9808, -104.5871) (10.067, -104.6142) (9.9924, -104.641) knots 0 0 0 0 1 1 1 1
  spline S1236 degree 3 poles (9.9924, -104.641) (9.9298, -104.6637) (9.9713, -104.6737) (10.0521, -104.6563) knots 0 0 0 0 1 1 1 1
  spline S1237 degree 3 poles (10.0521, -104.6563) (10.118, -104.6406) (10.1202, -104.6378) (10.0667, -104.6318) knots 0 0 0 0 1 1 1 1
  spline S1238 degree 3 poles (10.0667, -104.6318) (10.0132, -104.6258) (10.0153, -104.6231) (10.0813, -104.6074) knots 0 0 0 0 1 1 1 1
  spline S1239 degree 3 poles (10.0813, -104.6074) (10.1642, -104.5872) (10.2313, -104.6217) (10.1616, -104.6478) knots 0 0 0 0 1 1 1 1
  spline S1240 degree 3 poles (10.1616, -104.6478) (10.1353, -104.6586) (10.1359, -104.6636) (10.1641, -104.6676) knots 0 0 0 0 1 1 1 1
  spline S1241 degree 3 poles (10.1641, -104.6676) (10.1922, -104.6717) (10.23, -104.652) (10.2495, -104.627) knots 0 0 0 0 1 1 1 1
  spline S1242 degree 3 poles (10.2495, -104.627) (10.2821, -104.5853) (10.2877, -104.5896) (10.2817, -104.6431) knots 0 0 0 0 1 1 1 1
  spline S1243 degree 3 poles (10.2817, -104.6431) (10.2782, -104.6762) (10.2856, -104.6954) (10.2965, -104.6815) knots 0 0 0 0 1 1 1 1
  spline S1244 degree 3 poles (10.2965, -104.6815) (10.3182, -104.6537) (10.3228, -104.814) (10.32, -105.8146) knots 0 0 0 0 1 1 1 1
  spline S1245 degree 3 poles (10.32, -105.8146) (10.3214, -106.4604) (10.315, -106.5315) (10.2451, -106.5351) knots 0 0 0 0 1 1 1 1
  spline S1246 degree 3 poles (10.2451, -106.5351) (10.1773, -106.5359) (10.1773, -106.5359) (10.241, -106.5632) knots 0 0 0 0 1 1 1 1
  spline S1247 degree 3 poles (10.241, -106.5632) (10.3068, -106.5878) (10.317, -106.7524) (10.3184, -107.8279) knots 0 0 0 0 1 1 1 1
  spline S1248 degree 3 poles (10.3184, -107.8279) (10.3212, -108.5062) (10.3107, -109.0755) (10.2977, -109.0921) knots 0 0 0 0 1 1 1 1
  spline S1249 degree 3 poles (10.2977, -109.0921) (10.2825, -109.1116) (10.2363, -109.1248) (10.1912, -109.1253) knots 0 0 0 0 1 1 1 1
  spline S1250 degree 3 poles (10.1912, -109.1253) (10.1234, -109.1261) (10.129, -109.1304) (10.2174, -109.1548) knots 0 0 0 0 1 1 1 1
  spline S1251 degree 3 poles (10.2174, -109.1548) (10.2743, -109.1679) (10.3197, -109.19) (10.3209, -109.1999) knots 0 0 0 0 1 1 1 1
  spline S1252 degree 3 poles (10.3209, -109.1999) (10.3222, -109.2098) (10.3194, -109.7806) (10.3185, -110.4694) knots 0 0 0 0 1 1 1 1
  spline S1253 degree 3 poles (10.3185, -110.4694) (10.3176, -111.1581) (10.3196, -111.8088) (10.3197, -111.9118) knots 0 0 0 0 1 1 1 1
  spline S1254 degree 3 poles (10.3197, -111.9118) (10.3233, -112.0848) (10.3202, -112.1002) (10.2534, -112.0883) knots 0 0 0 0 1 1 1 1
  spline S1255 degree 3 poles (10.2534, -112.0883) (10.2125, -112.0833) (10.1841, -112.0969) (10.1865, -112.1167) knots 0 0 0 0 1 1 1 1
  spline S1256 degree 3 poles (10.1865, -112.1167) (10.1895, -112.1414) (10.2133, -112.1511) (10.2396, -112.1403) knots 0 0 0 0 1 1 1 1
  spline S1257 degree 3 poles (10.2396, -112.1403) (10.278, -112.1255) (10.2926, -112.1413) (10.3066, -112.215) knots 0 0 0 0 1 1 1 1
  spline S1258 degree 3 poles (10.3066, -112.215) (10.3213, -112.2936) (10.3295, -113.0566) (10.3154, -113.453) knots 0 0 0 0 1 1 1 1
  spline S1259 degree 3 poles (10.3154, -113.453) (10.3155, -113.5158) (10.3155, -113.8425) (10.3166, -114.1791) knots 0 0 0 0 1 1 1 1
  spline S1260 degree 3 poles (10.3166, -114.1791) (10.3187, -114.6061) (10.306, -114.7887) (10.2701, -114.783) knots 0 0 0 0 1 1 1 1
  spline S1261 degree 3 poles (10.2701, -114.783) (10.2447, -114.7811) (10.1803, -114.789) (10.1342, -114.8022) knots 0 0 0 0 1 1 1 1
  spline S1262 degree 3 poles (10.1342, -114.8022) (10.0562, -114.8218) (10.054, -114.8246) (10.1246, -114.826) knots 0 0 0 0 1 1 1 1
  spline S1263 degree 3 poles (10.1246, -114.826) (10.167, -114.8233) (10.2102, -114.8482) (10.2182, -114.8723) knots 0 0 0 0 1 1 1 1
  spline S1264 degree 3 poles (10.2182, -114.8723) (10.2296, -114.9036) (10.2367, -114.9002) (10.2402, -114.8671) knots 0 0 0 0 1 1 1 1
  spline S1265 degree 3 poles (10.2402, -114.8671) (10.2458, -114.8312) (10.2607, -114.8294) (10.282, -114.8595) knots 0 0 0 0 1 1 1 1
  spline S1266 degree 3 poles (10.282, -114.8595) (10.3048, -114.8818) (10.3201, -115.3951) (10.3188, -115.9985) knots 0 0 0 0 1 1 1 1
  spline S1267 degree 3 poles (10.3188, -115.9985) (10.3215, -117.4332) (10.3292, -117.3317) (10.2398, -117.3201) knots 0 0 0 0 1 1 1 1
  spline S1268 degree 3 poles (10.2398, -117.3201) (10.2011, -117.3123) (10.1726, -117.3258) (10.1757, -117.3506) knots 0 0 0 0 1 1 1 1
  spline S1269 degree 3 poles (10.1757, -117.3506) (10.1809, -117.3726) (10.1997, -117.3828) (10.2205, -117.3677) knots 0 0 0 0 1 1 1 1
  spline S1270 degree 3 poles (10.2205, -117.3677) (10.2413, -117.3526) (10.2706, -117.3666) (10.2864, -117.3923) knots 0 0 0 0 1 1 1 1
  spline S1271 degree 3 poles (10.2864, -117.3923) (10.3274, -117.4601) (10.3352, -119.5301) (10.2961, -119.5801) knots 0 0 0 0 1 1 1 1
  spline S1272 degree 3 poles (10.2961, -119.5801) (10.2831, -119.5968) (10.2854, -119.6568) (10.2983, -119.7206) knots 0 0 0 0 1 1 1 1
  spline S1273 degree 3 poles (10.2983, -119.7206) (10.3105, -119.7794) (10.3217, -120.3611) (10.3209, -121.0096) knots 0 0 0 0 1 1 1 1
  spline S1274 degree 3 poles (10.3209, -121.0096) (10.3185, -121.9524) (10.3074, -122.19) (10.2564, -122.2038) knots 0 0 0 0 1 1 1 1
  spline S1275 degree 3 poles (10.2564, -122.2038) (10.2096, -122.2121) (10.2053, -122.2176) (10.2446, -122.2304) knots 0 0 0 0 1 1 1 1
  spline S1276 degree 3 poles (10.2446, -122.2304) (10.2711, -122.2422) (10.2995, -122.2689) (10.3075, -122.293) knots 0 0 0 0 1 1 1 1
  spline S1277 degree 3 poles (10.3075, -122.293) (10.3241, -122.3463) (10.3229, -124.5882) (10.3056, -124.6105) knots 0 0 0 0 1 1 1 1
  spline S1278 degree 3 poles (10.3056, -124.6105) (10.2991, -124.6188) (10.3008, -124.6739) (10.3103, -124.7305) knots 0 0 0 0 1 1 1 1
  spline S1279 degree 3 poles (10.3103, -124.7305) (10.3225, -124.7894) (10.32, -124.8098) (10.3064, -124.7813) knots 0 0 0 0 1 1 1 1
  spline S1280 degree 3 poles (10.3064, -124.7813) (10.2929, -124.7528) (10.2878, -124.7936) (10.2982, -124.8778) knots 0 0 0 0 1 1 1 1
  spline S1281 degree 3 poles (10.2982, -124.8778) (10.3057, -124.9598) (10.3123, -125.0545) (10.3138, -125.087) knots 0 0 0 0 1 1 1 1
  spline S1282 degree 3 poles (10.3138, -125.087) (10.3087, -125.168) (10.2537, -125.2728) (10.2355, -125.2273) knots 0 0 0 0 1 1 1 1
  spline S1283 degree 3 poles (10.2355, -125.2273) (10.2282, -125.2081) (10.2052, -125.226) (10.1847, -125.2637) knots 0 0 0 0 1 1 1 1
  spline S1284 degree 3 poles (10.1847, -125.2637) (10.1642, -125.3014) (10.0166, -125.4502) (9.8535, -125.5959) knots 0 0 0 0 1 1 1 1
  spline S1285 degree 3 poles (9.8535, -125.5959) (9.559, -125.8582) (9.352, -126.0144) (9.3992, -125.9482) knots 0 0 0 0 1 1 1 1
  spline S1286 degree 3 poles (9.3992, -125.9482) (9.4116, -125.9266) (9.4213, -125.8626) (9.4168, -125.8053) knots 0 0 0 0 1 1 1 1
  spline S1287 degree 3 poles (9.4168, -125.8053) (9.4117, -125.7431) (9.4069, -125.6633) (9.4042, -125.6209) knots 0 0 0 0 1 1 1 1
  spline S1288 degree 3 poles (9.4042, -125.6209) (9.4015, -125.5785) (9.4081, -125.5299) (9.4212, -125.5133) knots 0 0 0 0 1 1 1 1
  spline S1289 degree 3 poles (9.4212, -125.5133) (9.4342, -125.4966) (9.4309, -125.4492) (9.4134, -125.4087) knots 0 0 0 0 1 1 1 1
  spline S1290 degree 3 poles (9.4134, -125.4087) (9.3958, -125.3681) (9.3959, -125.3279) (9.4101, -125.3211) knots 0 0 0 0 1 1 1 1
  spline S1291 degree 3 poles (9.4101, -125.3211) (9.4272, -125.3165) (9.4353, -125.2602) (9.4259, -125.2036) knots 0 0 0 0 1 1 1 1
  spline S1292 degree 3 poles (9.4259, -125.2036) (9.4024, -125.033) (9.398, -124.9355) (9.4119, -124.8032) knots 0 0 0 0 1 1 1 1
  spline S1293 degree 3 poles (9.4119, -124.8032) (9.421, -124.7342) (9.42, -124.6438) (9.4151, -124.6042) knots 0 0 0 0 1 1 1 1
  spline S1294 degree 3 poles (9.4151, -124.6042) (9.4075, -124.5624) (9.4122, -124.499) (9.4228, -124.4625) knots 0 0 0 0 1 1 1 1
  spline S1295 degree 3 poles (9.4228, -124.4625) (9.4341, -124.431) (9.432, -124.3935) (9.4181, -124.3827) knots 0 0 0 0 1 1 1 1
  spline S1296 degree 3 poles (9.4181, -124.3827) (9.4042, -124.3718) (9.3982, -124.2821) (9.4064, -124.1856) knots 0 0 0 0 1 1 1 1
  spline S1297 degree 3 poles (9.4064, -124.1856) (9.4229, -123.9925) (9.4211, -123.9777) (9.4067, -123.7784) knots 0 0 0 0 1 1 1 1
  spline S1298 degree 3 poles (9.4067, -123.7784) (9.4053, -123.7057) (9.4068, -123.5949) (9.4094, -123.5343) knots 0 0 0 0 1 1 1 1
  spline S1299 degree 3 poles (9.4094, -123.5343) (9.417, -123.473) (9.4156, -123.4003) (9.4048, -123.374) knots 0 0 0 0 1 1 1 1
  spline S1300 degree 3 poles (9.4048, -123.374) (9.394, -123.3477) (9.3991, -123.3068) (9.4143, -123.2874) knots 0 0 0 0 1 1 1 1
  spline S1301 degree 3 poles (9.4143, -123.2874) (9.4295, -123.2679) (9.4343, -123.2045) (9.422, -123.1457) knots 0 0 0 0 1 1 1 1
  spline S1302 degree 3 poles (9.422, -123.1457) (9.4125, -123.089) (9.4044, -123.0021) (9.4039, -122.9569) knots 0 0 0 0 1 1 1 1
  spline S1303 degree 3 poles (9.4039, -122.9569) (9.4055, -122.9089) (9.4018, -122.7762) (9.3999, -122.6583) knots 0 0 0 0 1 1 1 1
  spline S1304 degree 3 poles (9.3999, -122.6583) (9.3986, -122.5454) (9.4078, -122.4362) (9.4186, -122.4223) knots 0 0 0 0 1 1 1 1
  spline S1305 degree 3 poles (9.4186, -122.4223) (9.4295, -122.4084) (9.4334, -122.3174) (9.4246, -122.2255) knots 0 0 0 0 1 1 1 1
  spline S1306 degree 3 poles (9.4246, -122.2255) (9.4208, -122.133) (9.4161, -122.0129) (9.4199, -121.9622) knots 0 0 0 0 1 1 1 1
  spline S1307 degree 3 poles (9.4199, -121.9622) (9.4259, -121.9087) (9.4209, -121.8063) (9.4118, -121.732) knots 0 0 0 0 1 1 1 1
  spline S1308 degree 3 poles (9.4118, -121.732) (9.4027, -121.6577) (9.4081, -121.5992) (9.4229, -121.5974) knots 0 0 0 0 1 1 1 1
  spline S1309 degree 3 poles (9.4229, -121.5974) (9.435, -121.5934) (9.4307, -121.5587) (9.4154, -121.5154) knots 0 0 0 0 1 1 1 1
  spline S1310 degree 3 poles (9.4154, -121.5154) (9.395, -121.4727) (9.3951, -121.4324) (9.4143, -121.425) knots 0 0 0 0 1 1 1 1
  spline S1311 degree 3 poles (9.4143, -121.425) (9.4335, -121.4177) (9.4346, -121.3648) (9.4152, -121.3093) knots 0 0 0 0 1 1 1 1
  spline S1312 degree 3 poles (9.4152, -121.3093) (9.3958, -121.2539) (9.3935, -121.1939) (9.4087, -121.1744) knots 0 0 0 0 1 1 1 1
  spline S1313 degree 3 poles (9.4087, -121.1744) (9.4239, -121.155) (9.424, -121.1147) (9.4055, -121.0868) knots 0 0 0 0 1 1 1 1
  spline S1314 degree 3 poles (9.4055, -121.0868) (9.3891, -121.0562) (9.3861, -121.0314) (9.4009, -121.0296) knots 0 0 0 0 1 1 1 1
  spline S1315 degree 3 poles (9.4009, -121.0296) (9.413, -121.0256) (9.4196, -120.977) (9.4145, -120.9148) knots 0 0 0 0 1 1 1 1
  spline S1316 degree 3 poles (9.4145, -120.9148) (9.397, -120.731) (9.4006, -120.6175) (9.4254, -120.6144) knots 0 0 0 0 1 1 1 1
  spline S1317 degree 3 poles (9.4254, -120.6144) (9.4402, -120.6126) (9.4363, -120.5603) (9.4207, -120.4944) knots 0 0 0 0 1 1 1 1
  spline S1318 degree 3 poles (9.4207, -120.4944) (9.4029, -120.4312) (9.4023, -120.386) (9.4135, -120.3947) knots 0 0 0 0 1 1 1 1
  spline S1319 degree 3 poles (9.4135, -120.3947) (9.4246, -120.4034) (9.4262, -120.3555) (9.4149, -120.284) knots 0 0 0 0 1 1 1 1
  spline S1320 degree 3 poles (9.4149, -120.284) (9.4037, -120.2125) (9.4025, -120.1623) (9.4136, -120.171) knots 0 0 0 0 1 1 1 1
  spline S1321 degree 3 poles (9.4136, -120.171) (9.4248, -120.1797) (9.4249, -120.1395) (9.4126, -120.0807) knots 0 0 0 0 1 1 1 1
  spline S1322 degree 3 poles (9.4126, -120.0807) (9.4004, -120.0219) (9.4032, -119.9838) (9.4171, -119.9947) knots 0 0 0 0 1 1 1 1
  spline S1323 degree 3 poles (9.4171, -119.9947) (9.431, -120.0055) (9.4299, -119.9554) (9.4158, -119.8817) knots 0 0 0 0 1 1 1 1
  spline S1324 degree 3 poles (9.4158, -119.8817) (9.4018, -119.8081) (9.3978, -119.7558) (9.4117, -119.7666) knots 0 0 0 0 1 1 1 1
  spline S1325 degree 3 poles (9.4117, -119.7666) (9.4229, -119.7753) (9.4303, -119.7543) (9.431, -119.719) knots 0 0 0 0 1 1 1 1
  spline S1326 degree 3 poles (9.431, -119.719) (9.4296, -119.6865) (9.4494, -119.6439) (9.4752, -119.6281) knots 0 0 0 0 1 1 1 1
  spline S1327 degree 3 poles (9.4752, -119.6281) (9.5009, -119.6124) (9.5152, -119.5654) (9.5048, -119.5215) knots 0 0 0 0 1 1 1 1
  spline S1328 degree 3 poles (9.5048, -119.5215) (9.4885, -119.4506) (9.4836, -119.4512) (9.485, -119.5239) knots 0 0 0 0 1 1 1 1
  spline S1329 degree 3 poles (9.485, -119.5239) (9.4867, -119.579) (9.4759, -119.5929) (9.4536, -119.5755) knots 0 0 0 0 1 1 1 1
  spline S1330 degree 3 poles (9.4536, -119.5755) (9.4203, -119.5494) (9.3918, -119.4197) (9.4135, -119.3919) knots 0 0 0 0 1 1 1 1
  spline S1331 degree 3 poles (9.4135, -119.3919) (9.42, -119.3836) (9.4204, -119.3257) (9.4147, -119.2586) knots 0 0 0 0 1 1 1 1
  spline S1332 degree 3 poles (9.4147, -119.2586) (9.3999, -119.0769) (9.4007, -119.0014) (9.4221, -118.9913) knots 0 0 0 0 1 1 1 1
  spline S1333 degree 3 poles (9.4221, -118.9913) (9.432, -118.9901) (9.4287, -118.9427) (9.4099, -118.8922) knots 0 0 0 0 1 1 1 1
  spline S1334 degree 3 poles (9.4099, -118.8922) (9.3961, -118.8411) (9.3966, -118.7833) (9.4096, -118.7666) knots 0 0 0 0 1 1 1 1
  spline S1335 degree 3 poles (9.4096, -118.7666) (9.4248, -118.7472) (9.4258, -118.6942) (9.4154, -118.6503) knots 0 0 0 0 1 1 1 1
  spline S1336 degree 3 poles (9.4154, -118.6503) (9.4, -118.6069) (9.4023, -118.5639) (9.4165, -118.5572) knots 0 0 0 0 1 1 1 1
  spline S1337 degree 3 poles (9.4165, -118.5572) (9.4336, -118.5526) (9.4275, -118.503) (9.4109, -118.4498) knots 0 0 0 0 1 1 1 1
  spline S1338 degree 3 poles (9.4109, -118.4498) (9.3915, -118.3944) (9.3926, -118.3414) (9.4118, -118.3341) knots 0 0 0 0 1 1 1 1
  spline S1339 degree 3 poles (9.4118, -118.3341) (9.431, -118.3267) (9.4351, -118.2985) (9.4237, -118.2673) knots 0 0 0 0 1 1 1 1
  spline S1340 degree 3 poles (9.4237, -118.2673) (9.3948, -118.1954) (9.3895, -117.8869) (9.4179, -117.9538) knots 0 0 0 0 1 1 1 1
  spline S1341 degree 3 poles (9.4179, -117.9538) (9.4314, -117.9823) (9.4309, -117.9371) (9.415, -117.8486) knots 0 0 0 0 1 1 1 1
  spline S1342 degree 3 poles (9.415, -117.8486) (9.4019, -117.7623) (9.3989, -117.6973) (9.4128, -117.7081) knots 0 0 0 0 1 1 1 1
  spline S1343 degree 3 poles (9.4128, -117.7081) (9.4267, -117.719) (9.4314, -117.6958) (9.4216, -117.6568) knots 0 0 0 0 1 1 1 1
  spline S1344 degree 3 poles (9.4216, -117.6568) (9.4146, -117.62) (9.4098, -117.5401) (9.4146, -117.4767) knots 0 0 0 0 1 1 1 1
  spline S1345 degree 3 poles (9.4146, -117.4767) (9.4232, -117.3625) (9.4253, -117.3598) (9.5624, -117.3505) knots 0 0 0 0 1 1 1 1
  line L106 (9.5624, -117.3505) -> (9.6967, -117.339)
  line L107 (9.6967, -117.339) -> (9.5325, -117.3315)
  spline S1346 degree 3 poles (9.5325, -117.3315) (9.4443, -117.3298) (9.3818, -117.3123) (9.3949, -117.2957) knots 0 0 0 0 1 1 1 1
  spline S1347 degree 3 poles (9.3949, -117.2957) (9.4079, -117.279) (9.4161, -117.2227) (9.41, -117.1732) knots 0 0 0 0 1 1 1 1
  spline S1348 degree 3 poles (9.41, -117.1732) (9.3998, -117.0085) (9.4018, -116.9429) (9.4192, -116.9207) knots 0 0 0 0 1 1 1 1
  spline S1349 degree 3 poles (9.4192, -116.9207) (9.4301, -116.9068) (9.4268, -116.8595) (9.4135, -116.8133) knots 0 0 0 0 1 1 1 1
  spline S1350 degree 3 poles (9.4135, -116.8133) (9.4003, -116.7672) (9.4014, -116.7143) (9.4144, -116.6976) knots 0 0 0 0 1 1 1 1
  spline S1351 degree 3 poles (9.4144, -116.6976) (9.4296, -116.6782) (9.4254, -116.6435) (9.4118, -116.615) knots 0 0 0 0 1 1 1 1
  spline S1352 degree 3 poles (9.4118, -116.615) (9.3961, -116.5893) (9.3962, -116.5491) (9.4136, -116.5268) knots 0 0 0 0 1 1 1 1
  spline S1353 degree 3 poles (9.4136, -116.5268) (9.4288, -116.5074) (9.4316, -116.4693) (9.4187, -116.4458) knots 0 0 0 0 1 1 1 1
  spline S1354 degree 3 poles (9.4187, -116.4458) (9.4057, -116.4222) (9.3985, -116.3226) (9.4062, -116.2211) knots 0 0 0 0 1 1 1 1
  spline S1355 degree 3 poles (9.4062, -116.2211) (9.411, -116.1175) (9.4143, -116.0216) (9.4125, -116.0067) knots 0 0 0 0 1 1 1 1
  spline S1356 degree 3 poles (9.4125, -116.0067) (9.4003, -115.9479) (9.3932, -115.235) (9.4062, -115.2183) knots 0 0 0 0 1 1 1 1
  spline S1357 degree 3 poles (9.4062, -115.2183) (9.4192, -115.2016) (9.42, -115.1261) (9.4083, -114.9693) knots 0 0 0 0 1 1 1 1
  spline S1358 degree 3 poles (9.4083, -114.9693) (9.3993, -114.8548) (9.4079, -114.8436) (9.5482, -114.8189) knots 0 0 0 0 1 1 1 1
  line L108 (9.5482, -114.8189) -> (9.6664, -114.7993)
  line L109 (9.6664, -114.7993) -> (9.5324, -114.7932)
  line L110 (9.5324, -114.7932) -> (9.3957, -114.7848)
  line L111 (9.3957, -114.7848) -> (9.3973, -114.6338)
  spline S1359 degree 3 poles (9.3973, -114.6338) (9.3996, -114.5506) (9.4053, -114.4745) (9.414, -114.4634) knots 0 0 0 0 1 1 1 1
  spline S1360 degree 3 poles (9.414, -114.4634) (9.4205, -114.455) (9.4189, -114.3597) (9.4111, -114.2551) knots 0 0 0 0 1 1 1 1
  spline S1361 degree 3 poles (9.4111, -114.2551) (9.4033, -114.1505) (9.3978, -113.9627) (9.3996, -113.8343) knots 0 0 0 0 1 1 1 1